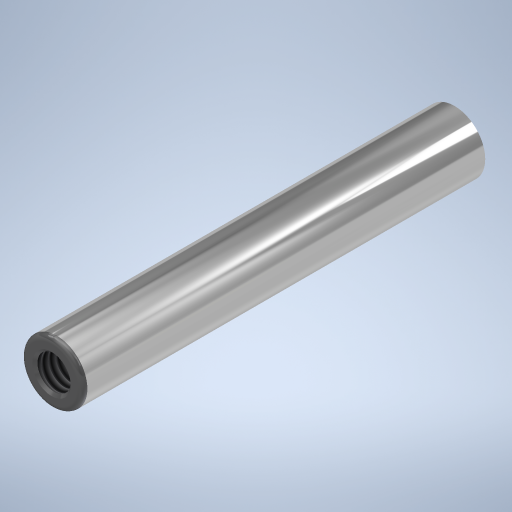
# Autodesk Inventor part: PIN, DOWEL, PULL, 6MMODX40MM
Saved by Autodesk Inventor 2024.2 (Build 282272000, 272)
## iProperties
Manager: 100-07519
Category: _
Material: Steel, 4140, Carb & Case Harden 58-60 Rc, 0.06 Dp Case
Document SubType Name: Modeling
Created: 2013-09-11
Designer: keithl , Keith
Manufacturer: Standard
Standards Organization: Custom
Checked By: 2FUS2
Engr Approved By: R
User Status: Released
Description: PIN, DOWEL, PULL, 6MMODX40MM
Density: 7.86 g/cm^3
Mass: 8.30101 g
Surface Area: 8.79367 cm^2
Volume: 1.05611 cm^3
Mfg Approved By: Keith.Leroux
Part Number: PIN, DOWEL, PULL, 6MMODX40MM
Appearance: Black Chrome
Control State: 0
Master: False
Checked Out: False
Shininess: 64.0
Angle Display Precision: 2
Document Length Units: 11269
Document Angle Units: 11279
Document Time Units: 11290
Document Mass Units: 11283
Document Length Units Precision: 3
Document Angle Units Precision: 2
CN_SERVICEABLE: _
FIRST_DESCRIPTION: PIN, DOWEL, PULL, 6MMODX40MM
PTC_WM_ITERATION: 6
PTC_WM_ORGANIZATION_ID: CLWC
PTC_WM_LIFECYCLE: CLWC_CAD_LC
CN_MASS: 0.008301
CL_runCount: 1
FinishProperty: ToBeSet
SECOND_DESCRIPTION: _
THIRD_DESCRIPTION: _
CN_MFG_PART_NUM: _
CUSTOMERNUMBER: _
Density: 0.0
Volumn: 0.0
Area: 0.0
PropertySet Name: Model Information
Revision Number: 1
Author: -
Keywords: -
Subject: _
Autodesk Inventor part; units mm, degrees
ref_plane "YZ Plane" through (0, 0, 0) normal (1, 0, 0) x (0, 1, 0)
ref_plane "XZ Plane" through (0, 0, 0) normal (0, 1, 0) x (-1, 0, 0)
ref_plane "XY Plane" through (0, 0, 0) normal (0, 0, 1) x (1, 0, 0)
sketch "Sketch1" plane through (0, 0, 0) normal (0, 0, 1) x (1, 0, 0)
  line L0 (0, 4.2) -> (0, -4.2) projected
  line L1 (-4.2, 0) -> (4.2, 0) projected
  circle A0 centre (0, 0) radius 3
  dimension "d0" = 6
  constraints: 1 centre point, 1 coincident
  measures "d0" diameter of A0
extrude "Extrusion1" add sketch "Sketch1" along normal mid plane 40
chamfer "Chamfer1" distance 1 angle 30 1 edges at (-3, 0, -20) measured on face at (-0.5351, 1.0949, -20)
fillet "Fillet1" radius 0.5 1 edges at (-3, 0, 20)
sketch "Sketch2" plane through (0, 0, 20) normal (0, 0, 1) x (1, 0, 0)
  circle A0 centre (0, 0) radius 2.5 projected
  constraints: 1 coincident
hole "Hole1" at (0, 0, 20) direction (0, 0, -1) diameter 3.242 depth 8 tip angle 118 thread size "M4x0.7" class "6H" standard "ANSI Metric M Profile"
chamfer "Chamfer2" distance 0.25 angle 45 1 edges at (0, 1.621, 20)
body "Solid1"
